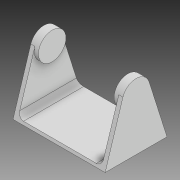
# Autodesk Inventor part: SpoolHolder
Saved by Autodesk Inventor 2020 (Build 240168000, 168)
## iProperties
Created: 2021-03-13
Part Number: SpoolHolder
Material: Generic
Document SubType Name: Modeling
Designer: DDeGo
Density: 1 g/cm^3
Appearance: Default
Author: DDeGo
Autodesk Inventor part; units mm, degrees
ref_plane "YZ Plane" through (0, 0, 0) normal (1, 0, 0) x (0, 1, 0)
ref_plane "XZ Plane" through (0, 0, 0) normal (0, 1, 0) x (-1, 0, 0)
ref_plane "XY Plane" through (0, 0, 0) normal (0, 0, 1) x (1, 0, 0)
sketch "Sketch1" plane through (0, 0, 0) normal (1, 0, 0) x (0, 1, 0)
  circle A0 centre (38, 0) radius 32 construction
  arc A1 (41.014111, -9.534943) -> (41.014111, 9.534943) centre (38, 0) ccw
  line L0 (41.014111, -9.534943) -> (0, -22.5)
  line L1 (0, -22.5) -> (0, 0)
  line L2 (0, 0) -> (28, 0) construction
  line L3 (41.014111, 9.534943) -> (0, 22.5)
  line L4 (0, 22.5) -> (0, 0)
  line L5 (38, 0) -> (28, 0) construction
  dimension "d0" = 20
  dimension "d1" = 64
  dimension "d2" = 38
  dimension "d3" = 45
  constraints: 12 end point, 2 centre point, 2 point on circle, 2 tangent, 2 vertical, 1 coincident, 1 equal length, 1 horizontal, 1 perpendicular
  measures "d0" diameter of A1
  measures "d1" diameter of A0
  measures "d2" distance from line of L1 A0.centre
  measures "d3" distance of L0.end L3.end
extrude "Extrusion1" add sketch "Sketch1" along normal blind 67
ref_plane "Work Plane1" through (0, 2, -22.5) normal (0, -1, 0) x (1, 0, 0)
sketch "Sketch2" plane through (0, 2, -22.5) normal (0, -1, 0) x (1, 0, 0)
  line L0 (0, 45) -> (0, 0) construction
  line L1 (0, 0) -> (67, 0) construction
  line L2 (67, 45) -> (67, 0) construction
  line L3 (0, 45) -> (67, 45) construction
  line L4 (0, 45) -> (67, 45) construction
  line L5 (0, 0) -> (67, 0) construction
  line L6 (64, 45) -> (3, 45)
  line L7 (3, 45) -> (3, 0)
  line L8 (3, 0) -> (64, 0)
  line L9 (64, 0) -> (64, 45)
  line L10 (67, 45) -> (67, 0) projected
  line L11 (67, 22.5) -> (64, 22.5) construction
  line L12 (0, 22.5) -> (3, 22.5) construction
  dimension "d7" = 61
  constraints: 12 end point, 3 midpoint, 2 parallel, 2 point on line, 1 collinear, 1 horizontal, 1 perpendicular
  measures "d7" distance between parallel lines of L7 L9
extrude "Extrusion2" cut sketch "Sketch2" against normal through all
sketch "Sketch3" plane through (3, 2, 21.867776) normal (1, 0, 0) x (0, 0, -1)
  arc A0 (31.402719, 39.014111) -> (12.332833, 39.014111) centre (21.867776, 36) ccw
  circle A1 centre (21.867776, 36) radius 10
  point P0 (21.867776, -2)
  constraints: 1 coincident, 3 other
extrude "Extrusion3" add sketch "Sketch3" along normal blind 3
sketch "Sketch4" plane through (64, 2, -21.867776) normal (-1, 0, 0) x (0, 0, 1)
  arc A0 (31.402719, 39.014111) -> (12.332833, 39.014111) centre (21.867776, 36) ccw
  circle A1 centre (21.867776, 36) radius 10
  point P0 (21.867776, -2)
  point P1 (12.332833, 39.014111)
  constraints: 1 coincident, 3 other
extrude "Extrusion4" add sketch "Sketch4" along normal blind 3
fillet "Fillet1" radius 4 2 edges at (64, 2, 0) (3, 2, 0)
body "Solid1"
